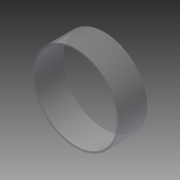
# Autodesk Inventor part: Bucketr
Saved by Autodesk Inventor 2013 (Build 170138000, 138)
## iProperties
Created: 2013-03-21
Part Number: Bucketr
Material: Polycarbonate, Clear
Document SubType Name: Modeling
Designer: actoennies
Mass: 725.889 g
Surface Area: 2024.3 cm^2
Volume: 604.907 cm^3
Density: 1.2 g/cm^3
Author: actoennies
Autodesk Inventor part; units mm, degrees
ref_plane "YZ Plane" through (0, 0, 0) normal (1, 0, 0) x (0, 1, 0)
ref_plane "XZ Plane" through (0, 0, 0) normal (0, 1, 0) x (-1, 0, 0)
ref_plane "XY Plane" through (0, 0, 0) normal (0, 0, 1) x (1, 0, 0)
sketch "Sketch1" plane through (0, 0, 0) normal (0, 0, 1) x (1, 0, 0)
  circle A0 centre (0, 0) radius 152.4
  circle A1 centre (0, 0) radius 146.05
  dimension "d0" = 304.8
  dimension "d1" = 292.1
  constraints: 2 centre point, 2 coincident
  measures "d0" diameter of A0
  measures "d1" diameter of A1
extrude "Extrusion1" add sketch "Sketch1" along normal blind 101.6
sketch "Sketch2" plane through (0, 0, 101.6) normal (0, 0, 1) x (1, 0, 0)
  circle A0 centre (0, 0) radius 146.05 projected
  circle A1 centre (0, 0) radius 152.4 projected
  line L0 (0, -146.05) -> (0, -152.4)
  line L1 (0, 146.05) -> (0, 152.4)
  constraints: 4 end point, 4 point on circle, 1 collinear, 1 vertical
extrude "Extrusion3" cut sketch "Sketch2" against normal blind 38.1 contours A0 L0 A1 L1 picked at (-148.0019, 0)
ref_plane "Work Plane1" through (152.4, 0, 0) normal (-1, 0, 0) x (0, -1, 0)
sketch "Sketch3" plane through (152.4, 0, 0) normal (-1, 0, 0) x (0, -1, 0)
  line L0 (-4.7625, 101.6) -> (-4.7625, 76.2)
  line L1 (-4.7625, 76.2) -> (-23.8125, 76.2)
  line L2 (-23.8125, 76.2) -> (-23.8125, 101.6)
  line L3 (-23.8125, 101.6) -> (-4.7625, 101.6)
  line L4 (-152.4, 0) -> (152.4, 0) projected
  point P0 (0, 0)
  dimension "d8" = 25.4
  dimension "d9" = 19.05
  dimension "d10" = 4.7625
  dimension "d11" = 101.6
  constraints: 8 end point, 2 parallel, 1 perpendicular, 1 vertical
  measures "d8" distance of L0.start L0.end
  measures "d9" distance of L0.end L1.end
  measures "d10" distance from line of point (0, 0) L0
  measures "d11" distance between parallel lines of L4 L3
extrude "Extrusion4" cut sketch "Sketch3" along normal blind 38.1
body "Solid1"
